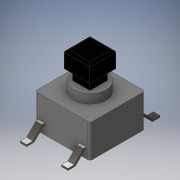
# Autodesk Inventor part: TL3301SPF160QG_Tactile
Saved by Autodesk Inventor 2016 (Build 200138000, 138)
## iProperties
Created: 2016-09-23
Part Number: TL3301SPF160QG_Tactile
Material: Generic
Document SubType Name: Modeling
Designer: jfixelle
Density: 1 g/cm^3
Appearance: Gray
Author: jfixelle
Autodesk Inventor part; units mm, degrees
ref_plane "XZ Plane" through (0, 0, 0) normal (0, 1, 0) x (-1, 0, 0)
ref_plane "XY Plane" through (0, 0, 0) normal (0, 0, 1) x (1, 0, 0)
sketch "Sketch1" plane through (0, 0, 0) normal (0, 1, 0) x (-1, 0, 0)
  line L0 (3, 3) -> (-3, 3)
  line L1 (-3, 3) -> (-3, -3)
  line L2 (-3, -3) -> (3, -3)
  line L3 (3, -3) -> (3, 3)
  point P0 (0, 0)
  dimension "d0" = 6
  dimension "d1" = 6
  dimension "d2" = 3
  dimension "d3" = 3
  constraints: 8 end point, 2 parallel, 1 horizontal, 1 perpendicular
  measures "d0" distance of L2.end L0.start
  measures "d1" distance of L1.end L2.end
  measures "d2" distance from line of point (0, 0) L2
  measures "d3" distance from line of point (0, 0) L3
extrude "Extrusion1" add sketch "Sketch1" along normal blind 3.6
fillet "Fillet1" radius 0.25 4 edges at (3, 1.8, 3) (3, 1.8, -3) (-3, 1.8, 3) (-3, 1.8, -3)
sketch "Sketch2" plane through (0, 3.6, 0) normal (0, 1, 0) x (1, 0, 0)
  circle A0 centre (0, 0) radius 1.75
  dimension "d7" = 3.5
  constraints: 1 centre point, 1 coincident
  measures "d7" diameter of A0
extrude "Extrusion2" add sketch "Sketch2" along normal blind 1
sketch "Sketch3" plane through (0, 4.6, 0) normal (0, 1, 0) x (1, 0, 0)
  line L0 (0.95, -0.95) -> (-0.95, -0.95)
  line L1 (-0.95, -0.95) -> (-0.95, 0.95)
  line L2 (-0.95, 0.95) -> (0.95, 0.95)
  line L3 (0.95, 0.95) -> (0.95, -0.95)
  point P0 (0, 0)
  dimension "d10" = 1.9
  dimension "d11" = 1.9
  dimension "d12" = 0.95
  dimension "d13" = 0.95
  constraints: 8 end point, 2 parallel, 1 horizontal, 1 perpendicular
  measures "d10" distance of L0.end L1.end
  measures "d11" distance of L1.end L2.end
  measures "d12" distance from line of point (0, 0) L1
  measures "d13" distance from line of point (0, 0) L2
extrude "Extrusion3" add sketch "Sketch3" along normal blind 1.1
sketch "Sketch4" plane through (0, 5.7, 0) normal (0, 1, 0) x (1, 0, 0)
  line L0 (-1.4, -1.4) -> (1.4, -1.4)
  line L1 (1.4, -1.4) -> (1.4, 1.4)
  line L2 (1.4, 1.4) -> (-1.4, 1.4)
  line L3 (-1.4, 1.4) -> (-1.4, -1.4)
  point P0 (0, 0)
  dimension "d16" = 2.8
  dimension "d17" = 2.8
  dimension "d18" = 1.4
  dimension "d19" = 1.4
  constraints: 8 end point, 2 parallel, 1 horizontal, 1 perpendicular
  measures "d16" distance of L2.end L0.start
  measures "d17" distance of L1.end L2.end
  measures "d18" distance from line of point (0, 0) L3
  measures "d19" distance from line of point (0, 0) L2
extrude "Extrusion4" add sketch "Sketch4" along normal blind 1.8
fillet "Fillet2" radius 0.25 4 edges at (1.4, 7.5, 0) (0, 7.5, 1.4) (-1.4, 7.5, 0) (0, 7.5, -1.4)
ref_plane "Work Plane1" through (2.25, 0, 0) normal (1, 0, 0) x (0, 1, 0)
sketch "Sketch5" plane through (2.25, 0, 0) normal (1, 0, 0) x (0, 1, 0)
  line L0 (1.1258, -3.3032) -> (1.1258, -2.4976)
  line L1 (1.1258, -2.4976) -> (0.9258, -2.4976)
  line L2 (0.9258, -2.4976) -> (0.9258, -3.1742)
  line L3 (0.9258, -3.1742) -> (-0.1, -4.2)
  line L4 (-0.1, -4.2) -> (-0.1, -5)
  line L5 (-0.1, -5) -> (0.1, -5)
  line L6 (0.1, -5) -> (0.1, -4.329)
  line L7 (0.1, -4.329) -> (1.1258, -3.3032)
  line L8 (0, 0) -> (-0.9994, 0)
  line L9 (0, 2.75) -> (0, -2.75) projected
  dimension "d24" = 4.2
  dimension "d25" = 5
  dimension "d26" = 0.1
  dimension "d27" = 0.2
  dimension "d28" = 0.2
  dimension "d29" = 45
  dimension "d30" = 45
  constraints: 18 end point, 4 perpendicular, 1 horizontal, 1 parallel, 1 vertical
  measures "d24" distance from line of L3.end L8
  measures "d25" distance between parallel lines of L5 L8
  measures "d26" distance between parallel lines of L4 L9
  measures "d27" distance of L4.end L5.end
  measures "d28" distance between parallel lines of L2 L0
  measures "d29" angle of L4 L3
  measures "d30" angle of L6 L7
extrude "Extrusion5" add sketch "Sketch5" along normal mid plane 0.7
mirror "Mirror1" about plane through (0, 0, 0) normal (1, 0, 0) of "Extrusion5"
mirror "Mirror2" about plane through (0, 0, 0) normal (0, 0, 1) of "Extrusion5", "Mirror1"
body "Solid1"
